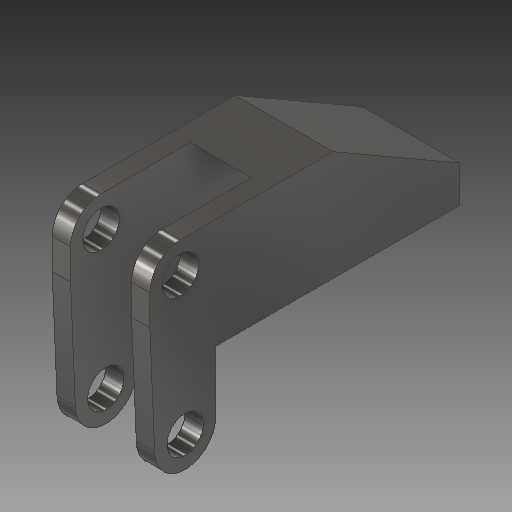
# Autodesk Inventor part: Finger
Saved by Autodesk Inventor 2019 (Build 230136000, 136)
## iProperties
Created: 2018-12-28
Part Number: Finger
Material: 钢，高强度，低合金
Document SubType Name: Modeling
Designer: JianQiao Hu
Density: 7.85 g/cm^3
Appearance: 钢 - 抛光
Author: JianQiao Hu
Autodesk Inventor part; units mm, degrees
ref_plane "YZ Plane" through (0, 0, 0) normal (1, 0, 0) x (0, 1, 0)
ref_plane "XZ Plane" through (0, 0, 0) normal (0, 1, 0) x (-1, 0, 0)
sketch "草图1" plane through (0, 0, 0) normal (1, 0, 0) x (0, 1, 0)
  circle A0 centre (0, 0) radius 15
  arc A1 (0, 25) -> (0, -25) centre (0, 0) ccw
  line L0 (0, -25) -> (50, -25)
  line L1 (50, -25) -> (50, -225)
  line L2 (50, -225) -> (80, -225)
  line L3 (80, -225) -> (140, -121.077)
  line L4 (140, -121.077) -> (140, 28.923)
  line L5 (140, 28.923) -> (90, 28.923)
  line L6 (90, 28.923) -> (0, 25)
  dimension "d0" = 30
  dimension "d1" = 50
  dimension "d2" = 50
  dimension "d4" = 200
  dimension "d5" = 30
  dimension "d6" = 30
  dimension "d7" = 120
  dimension "d8" = 150
  dimension "d9" = 50
  constraints: 14 end point, 3 perpendicular, 2 centre point, 2 coincident, 2 point on circle, 1 horizontal, 1 parallel, 1 tangent
  measures "d0" diameter of A0
  measures "d1" diameter of A1
  measures "d2" distance of L0.start L0.end
  measures "d4" distance of L0.end L1.end
  measures "d5" distance of L1.end L2.end
  measures "d6" angle of L1 L3
  measures "d7" distance of L2.end L3.end
  measures "d8" distance of L3.end L4.end
  measures "d9" distance of L4.end L5.end
extrude "拉伸1" add sketch "草图1" along normal mid plane 80
sketch "草图2" plane through (-40, 50, -225) normal (0, -1, 0) x (1, 0, 0)
  line L0 (80, 0) -> (0, 0) projected
  line L1 (40, 0) -> (40, 253.923)
  line L2 (80, 253.923) -> (0, 253.923) projected
  line L3 (15, -693.1323) -> (65, -693.1323)
  line L4 (65, -693.1323) -> (65, 466.9493)
  line L5 (65, 466.9493) -> (15, 466.9493)
  line L6 (15, 466.9493) -> (15, -693.1323)
  line L7 (15, -693.1323) -> (65, 466.9493) construction
  line L8 (65, -693.1323) -> (15, 466.9493) construction
  point P0 (40, 225)
  point P1 (40, -113.0915)
  dimension "d12" = 50
  constraints: 14 end point, 4 midpoint, 2 parallel, 1 horizontal, 1 perpendicular, 1 point on line
  measures "d12" distance of L4.end L5.end
extrude "拉伸2" cut sketch "草图2" along normal through all
ref_plane "工作平面2" through (0, 50, 27.1795) normal (0, 0.8660254, -0.5) x (1, 0, 0)
sketch "草图3" plane through (0, 50, 27.1795) normal (0, 0.8660254, -0.5) x (1, 0, 0)
  line L0 (25, -307.1385) -> (-25, -307.1385)
  line L1 (-25, -307.1385) -> (-25, 307.1385)
  line L2 (-25, 307.1385) -> (25, 307.1385)
  line L3 (25, 307.1385) -> (25, -307.1385)
  line L4 (-25, 0) -> (25, 0) projected
  line L5 (25, -307.1385) -> (-25, 307.1385) construction
  line L6 (-25, -307.1385) -> (25, 307.1385) construction
  point P0 (0, 48.5381)
  point P1 (0, 0)
  dimension "d16" = 50
  constraints: 12 end point, 3 midpoint, 2 parallel, 1 horizontal, 1 perpendicular
  measures "d16" distance of L0.start L0.end
extrude "拉伸3" cut sketch "草图3" along normal up to surface (126.0897 mm away)
fillet "圆角1" radius 25 2 edges at (-32.5, 140, 28.923) (32.5, 140, 28.923)
sketch "草图4" plane through (-40, 0, 0) normal (-1, 0, 0) x (0, 0, 1)
  line L0 (3.923, 140) -> (-121.077, 140) projected
  line L1 (28.923, 90) -> (28.923, 115) projected
  point P0 (0, 0)
  point P1 (3.923, 115)
  dimension "d27" = 25
  dimension "d28" = 25
  measures "d27" distance from line of L0 point (3.923, 115)
  measures "d28" distance from line of L1 point (3.923, 115)
hole "孔1" at (-40, 115, 3.923) direction (1, 0, 0) diameter 30 end through all
sketch "草图5" plane through (25, 0, -25) normal (-1, 0, 0) x (0, 0, 1)
  point P0 (25, 0)
